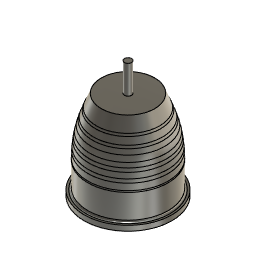
Lampe_R1 v11 (Autodesk Fusion 360 archive; units mm, degrees)
design "Cobstaled MR16"
Autodesk Fusion 360 part; units mm, degrees
sketch "Skizze1" plane through (0, 0, 0) normal (0, 0, 1) x (1, 0, 0)
  circle A0 centre (0, 0) radius 24.75
  circle A1 centre (0, 0) radius 20
  dimension "d1" = 49.5
  dimension "d4" = 40
  constraint coincident A0.centre A1.centre
  measures "d1" diameter of A0
  measures "d4" diameter of A1
extrude "Extrusion1" add sketch "Skizze1" along normal blind 2.9
sketch "Skizze2" plane through (0, 0, 0) normal (0, 1, 0) x (1, 0, 0)
  line L0 (-24.75, -2.9) -> (24.75, -2.9)
  line L1 (-24.75, 0) -> (24.75, 0)
  line L2 (22.65, -2.9) -> (22.65, -7.9)
  line L3 (22.65, -7.9) -> (22.65, -12.9)
  line L4 (22.65, -12.9) -> (22.65, -17.9)
  line L5 (22.65, -17.9) -> (22.5, -22.8977)
  line L6 (22.5, -22.8977) -> (22, -27.8727)
  line L7 (22, -27.8727) -> (21.15, -32.7999)
  line L8 (21.15, -32.7999) -> (19.75, -37.5999)
  line L9 (19.75, -37.5999) -> (18.1, -42.3198)
  line L10 (0, -2.9) -> (0, -41.75) construction
  line L11 (18.1, -42.3198) -> (15.05, -49.9)
  line L12 (15.05, -49.9) -> (0, -49.9)
  line L13 (0, -49.9) -> (0, -2.9)
  dimension "d6" = 5
  dimension "d8" = 22.65
  dimension "d9" = 22.65
  dimension "d10" = 22.65
  dimension "d11" = 22.65
  dimension "d12" = 22.5
  dimension "d13" = 22
  dimension "d14" = 21.15
  dimension "d15" = 19.75
  dimension "d17" = 18.1
  dimension "d18" = 47
  dimension "d20" = 15.05
  dimension "d21" = 8.1708
  dimension "d22" = 7.5802
  constraint coincident L0 L2.start
  constraint equal L2 L3
  constraint equal L2 L4
  constraint equal L2 L5
  constraint equal L2 L6
  constraint equal L2 L7
  constraint equal L2 L8
  constraint equal L2 L9
  constraint midpoint L0 L10.start
  constraint perpendicular L0 L10
  constraint vertical L10.end L12.end
  constraint perpendicular L10 L12
  measures "d6" distance of L2.start L2.end
  measures "d8" distance of L2.end L10
  measures "d9" distance of L2.start L10
  measures "d10" distance of L3.end L10
  measures "d11" distance of L4.end L10
  measures "d12" distance of L5.end L10
  measures "d13" distance of L6.end L10
  measures "d14" distance of L7.end L10
  measures "d15" distance of L8.end L10
  measures "d17" distance of L9.end L10
  measures "d18" distance of L0 L11.end
  measures "d20" distance of L10 L11.end
  measures "d21" distance of L9.end L11.end
  measures "d22" distance of L9.end L12
revolve "Drehen1" add sketch "Skizze2" angle 360 about axis through (0, 0, 49.9) along (0, 0, -1)
fillet "Abrundung1" radius 28 6 edges at (-16.8751, -6.5452, 42.3198) (-18.4135, -7.1419, 37.5999) (-19.7187, -7.6482, 32.7999) (-20.5112, -7.9555, 27.8727) (-20.9774, -8.1363, 22.8977) (-21.1172, -8.1906, 17.9)
fillet "Abrundung2" radius 1 1 edges at (-21.1172, 8.1906, 2.9)
sketch "Skizze3" plane through (0, 0, 49.9) normal (0, 0, 1) x (-1, 0, 0)
  circle A0 centre (0, 0) radius 15.05
  circle A1 centre (0, 0) radius 2
  dimension "d28" = 4
  constraint coincident A0.centre A1.centre
  measures "d28" diameter of A1
extrude "Extrusion2" add sketch "Skizze3" along normal blind 16 contours A1
equation "d8 = ( 45.3 / 2 ) * 1 mm"
equation "d9 = ( 45.3 / 2 ) * 1 mm"
equation "d10 = ( 45.3 / 2 ) * 1 mm"
equation "d11 = ( 45.3 / 2 ) * 1 mm"
equation "d12 = ( 45.0 / 2 ) * 1 mm"
equation "d13 = ( 44 / 2 ) * 1 mm"
equation "d14 = ( 42.3 / 2 ) * 1 mm"
equation "d15 = ( 39.5 / 2 ) * 1 mm"
equation "d17 = ( 36.2 / 2 ) * 1 mm"
equation "d20 = ( 30.1 / 2 ) * 1 mm"
